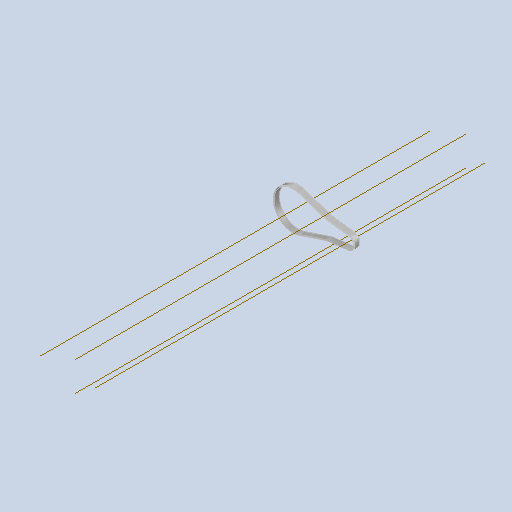
# Autodesk Inventor part: Synchronous Belt
Saved by Autodesk Inventor 2022.2 (Build 262287030, 287C)
## iProperties
CustomPartVersion: 1
Created: 2022-01-04
Part Number: Synchronous Belt
Material: Rubber
Document SubType Name: Modeling
Designer: Jochen
Density: 1 g/cm^3
Appearance: Rubber - Black - Version 1.1
Author: Jochen
Autodesk Inventor part; units mm, degrees
ref_plane "YZ Plane" through (0, 0, 0) normal (1, 0, 0) x (0, 1, 0)
ref_plane "XZ Plane" through (0, 0, 0) normal (0, 1, 0) x (-1, 0, 0)
ref_plane "XY Plane" through (0, 0, 0) normal (0, 0, 1) x (1, 0, 0)
sketch "Sketch Path" plane through (0, 0, 0) normal (0, 0, 1) x (1, 0, 0)
  arc A0 (0.57762, -4.73958) -> (0.57762, 4.73958) centre (0, 0) ccw
  arc A1 (-15.425411, -6.689896) -> (-16.248049, -6.873367) centre (-14.905212, -10.958314) ccw
  arc A2 (-36.733687, 13.60757) -> (-36.733687, -13.60757) centre (-41.206876, 0) ccw
  arc A3 (-16.248049, 6.873367) -> (-15.425411, 6.689896) centre (-14.905212, 10.958314) ccw
  line L0 (-15.425411, 6.689896) -> (0.57762, 4.73958)
  line L1 (0.57762, -4.73958) -> (-15.425411, -6.689896)
  line L2 (-16.248049, -6.873367) -> (-36.733687, -13.60757)
  line L3 (-36.733687, 13.60757) -> (-16.248049, 6.873367)
  constraints: 8 end point, 8 point on circle, 4 centre point
ref_plane "Cross Section Plane" through (0.57762, 4.73958, 0) normal (-0.9926554, 0.1209765, 0) x (0, 0, 1)
ref_plane "Work Plane2" through (0, 0, 0) normal (-1, 0, 0) x (0, 0, 1)
ref_plane "Work Plane3" through (-41.206876, 0, 0) normal (0.950674, 0.3101917, 0) x (0, 0, 1)
sketch "Cross Section" plane through (0.57762, 4.73958, 0) normal (-0.9926554, 0.1209765, 0) x (0, 0, 1)
  line L0 (-2, 0.3) -> (2, 0.3)
  line L1 (2, 0.3) -> (2, -0.3)
  line L2 (2, -0.3) -> (-2, -0.3)
  line L3 (-2, -0.3) -> (-2, 0.3)
  line L4 (-2, 0) -> (2, 0) construction
  point P0 (0, 0)
  point P1 (0, 0)
  dimension "d0" = 4
  dimension "d4" = 0.3
  dimension "d5" = 0.3
  constraints: 10 end point, 3 midpoint, 2 parallel, 1 coincident, 1 horizontal, 1 perpendicular, 1 other
  measures "d0" distance between parallel lines of L1 L3
  measures "d4" distance between parallel lines of L2 L4
  measures "d5" distance between parallel lines of L4 L0
sweep "Belt" add profiles "Cross Section" path "Sketch Path" path curves L3 A3 L0 A0 L1 A1 L2 A2
equation "\"d0\" = da_B"
equation "\"d4\" = da_a"
equation "\"d5\" = da_a2"
equation "\"da_B\" = 4"
equation "\"da_pb\" = 2.5"
equation "\"da_L\" = 145"
equation "\"da_a\" = 0.3"
equation "\"da_S\" = 1.5"
equation "\"da_Beta\" = 20deg"
equation "\"da_Ht\" = 0.7"
equation "\"da_H\" = 1.3"
equation "\"da_a2\" = 0.3"
body "Solid1"
